lower arm (Autodesk Fusion 360 design; units mm, degrees)
Autodesk Fusion 360 part; units mm, degrees
sketch "Sketch1" plane through (0, 0, 28.25) normal (0, 0, -1) x (1, 0, 0)
  circle A0 centre (0, -70.5) radius 2.95
  circle A1 centre (0, -20.5) radius 4.05
  arc A2 (-5, -70.5) -> (5, -70.5) centre (0, -70.5) ccw
  line L0 (5, -70.5) -> (5, -23.8166)
  arc A3 (5, -23.8166) -> (-5, -23.8166) centre (0, -20.5) ccw
  line L1 (-5, -23.8166) -> (-5, -70.5)
  circle A4 centre (0, -70.5) radius 3.05
  circle A5 centre (0, -70.5) radius 6
  line L2 (0, -70.5) -> (-40, -70.5) construction
  line L3 (0, -70.5) -> (20, -70.5) construction
  circle A6 centre (20, -70.5) radius 5
  circle A7 centre (-40, -70.5) radius 5
  line L4 (-40.125, -65.5016) -> (-0.15, -64.5019)
  line L5 (-40.125, -75.4984) -> (-0.15, -76.4981)
  line L6 (0.3, -76.4925) -> (20.25, -75.4937)
  line L7 (0.3, -64.5075) -> (20.25, -65.5063)
  dimension "d155" = 6.1
  dimension "d156" = 12
  dimension "d157" = 40
  dimension "d158" = 20
  dimension "d159" = 10
  dimension "d160" = 10
  constraint concentric A0 A4
  constraint concentric A4 A5
  constraint coincident A0.centre A2.centre
  constraint horizontal L2
  constraint parallel L2 L3
  constraint coincident L3.end A6.centre
  constraint coincident L2.end A7.centre
  constraint coincident A7 L4.start
  constraint coincident A5 L4.end
  constraint tangent A5 L4
  constraint coincident A7 L5.start
  constraint coincident A5 L5.end
  constraint tangent A5 L5
  constraint coincident A5 L6.start
  constraint coincident A6 L6.end
  constraint tangent A6 L6
  constraint coincident A5 L7.start
  constraint coincident A6 L7.end
  constraint tangent A6 L7
  constraint tangent A5 L7
  constraint tangent A5 L6
  constraint tangent A7 L5
  constraint tangent A7 L4
  measures "d155" diameter of A4
  measures "d156" diameter of A5
  measures "d157" distance of A0.centre L2.end
  measures "d158" distance of A0.centre L3.end
  measures "d159" diameter of A6
  measures "d160" diameter of A7
extrude "Extrude1" add sketch "Sketch1" along normal blind 7 contours A2 L0 L1 A5 | A2 L0 L1 A5 | L1 A5 A7 L4 L5 | L1 A5 L4 | L0 A5 L7 | L0 A5 A6 L6 L7 | A7 | A6 makes body 1
sketch "Sketch2" plane through (0, 0, 28.25) normal (0, 0, 1) x (-1, 0, 0)
  circle A0 centre (0, -70.5) radius 3.05
  arc A1 (40.125, -75.4984) -> (40.125, -65.5016) centre (40, -70.5) ccw
  line L0 (40.125, -65.5016) -> (0.15, -64.5019)
  arc A2 (0.15, -64.5019) -> (-0.3, -64.5075) centre (0, -70.5) ccw
  line L1 (-0.3, -64.5075) -> (-20.25, -65.5063)
  arc A3 (-20.25, -65.5063) -> (-20.25, -75.4937) centre (-20, -70.5) ccw
  line L2 (-20.25, -75.4937) -> (-0.3, -76.4925)
  arc A4 (-0.3, -76.4925) -> (0.15, -76.4981) centre (0, -70.5) ccw
  line L3 (0.15, -76.4981) -> (40.125, -75.4984)
  circle A5 centre (-20, -70.5) radius 2.95
  dimension "d175" = 5.9
  constraint concentric A3 A5
  measures "d175" diameter of A5
extrude "Extrude2" add sketch "Sketch2" along normal blind 4 contours A5 bodies 1
extrude "Extrude3" add 1 faces at (21.1585, 69.8312, 32.25) along direction (0, 0, 1) blind 1 on bodies 1 bodies 1
extrude "Extrude4" cut 1 faces at (21.1585, 69.8312, 33.25) along direction (0, 0, -1) blind 5 on bodies 1 bodies 1
sketch "Sketch3" plane through (0, 0, 28.25) normal (0, 0, 1) x (-1, 0, 0)
  circle A0 centre (0, -70.5) radius 3.05
  arc A1 (40.125, -75.4984) -> (40.125, -65.5016) centre (40, -70.5) ccw
  line L0 (40.125, -65.5016) -> (0.15, -64.5019)
  arc A2 (0.15, -64.5019) -> (-0.3, -64.5075) centre (0, -70.5) ccw
  line L1 (-0.3, -64.5075) -> (-20.25, -65.5063)
  arc A3 (-20.25, -65.5063) -> (-20.25, -75.4937) centre (-20, -70.5) ccw
  line L2 (-20.25, -75.4937) -> (-0.3, -76.4925)
  arc A4 (-0.3, -76.4925) -> (0.15, -76.4981) centre (0, -70.5) ccw
  line L3 (0.15, -76.4981) -> (40.125, -75.4984)
  circle A5 centre (-20, -70.5) radius 1.25
  dimension "d216" = 2.5
  constraint concentric A3 A5
  measures "d216" diameter of A5
extrude "Extrude5" cut sketch "Sketch3" against normal blind 2 contours A5 bodies 1
extrude "Extrude6" cut 1 faces at (19.6557, 70.1411, 26.25) along direction (0, 0, -1) blind 0.8 draft 45 on bodies 1 bodies 1
extrude "Extrude7" cut 1 faces at (19.3243, 70.6018, 25.45) along direction (0, 0, -1) up to surface (4.2 mm away) on bodies 1 bodies 1
sketch "Sketch4" plane through (0, 0, 28.25) normal (0, 0, 1) x (-1, 0, 0)
  circle A0 centre (-20, -70.5) radius 1.25
  circle A1 centre (0, -70.5) radius 3.05
  arc A2 (40.125, -75.4984) -> (40.125, -65.5016) centre (40, -70.5) ccw
  line L0 (40.125, -65.5016) -> (0.15, -64.5019)
  arc A3 (0.15, -64.5019) -> (-0.3, -64.5075) centre (0, -70.5) ccw
  line L1 (-0.3, -64.5075) -> (-20.25, -65.5063)
  arc A4 (-20.25, -65.5063) -> (-20.25, -75.4937) centre (-20, -70.5) ccw
  line L2 (-20.25, -75.4937) -> (-0.3, -76.4925)
  arc A5 (-0.3, -76.4925) -> (0.15, -76.4981) centre (0, -70.5) ccw
  line L3 (0.15, -76.4981) -> (40.125, -75.4984)
  line L4 (40, -70.5) -> (30.0031, -70.25) construction
  circle A6 centre (30.0031, -70.25) radius 3
  line L5 (32.1275, -65.3016) -> (31.8673, -75.7049)
  dimension "d250" = 10
  dimension "d251" = 6
  dimension "d252" = 2
  constraint coincident A2.centre L4.start
  constraint parallel L0 L4
  constraint coincident L4.end A6.centre
  constraint coincident L0 L5.start
  constraint coincident L3 L5.end
  constraint perpendicular L4 L5
  measures "d250" distance of A2.centre L4.end
  measures "d251" diameter of A6
  measures "d252" distance of L4.end L5
extrude "Extrude8" cut sketch "Sketch4" against normal blind 7 contours A2 L0 L3 A6 L5 | A6 L5 | A6 L5 bodies 1
fillet "Fillet1" radius 0.25 2 edges at (-31.9466, 72.5354, 24.75) (-32.0584, 68.0646, 24.75) on bodies 1
extrude "Extrude9" add sketch "Sketch4" against normal blind 7 separate body contours A2 L0 L3 A6 L5 | A6 L5 | A6 L5 makes body 2
